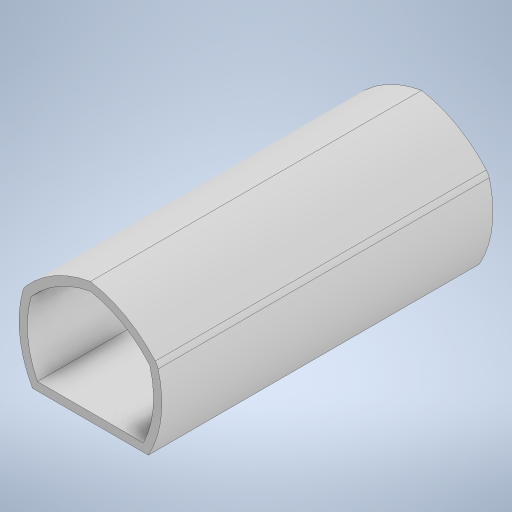
# Autodesk Inventor part: body
Saved by Autodesk Inventor 2024 (Build 280153000, 153)
## iProperties
Created: 2023-06-07
Part Number: body
Material: Generic
Document SubType Name: Modeling
Designer: tamiz
Density: 1 g/cm^3
Appearance: Default
Author: tamiz
Autodesk Inventor part; units mm, degrees
ref_plane "YZ Plane" through (0, 0, 0) normal (1, 0, 0) x (0, 1, 0)
ref_plane "XZ Plane" through (0, 0, 0) normal (0, 1, 0) x (-1, 0, 0)
ref_plane "XY Plane" through (0, 0, 0) normal (0, 0, 1) x (1, 0, 0)
sketch "Sketch3" plane through (0, 0, 0) normal (0, 0, 1) x (1, 0, 0)
  line L0 (3200.4, -3619.5) -> (-3200.4, -3619.5)
  line L1 (0, -3619.5) -> (0, 3086.1) construction
  arc A0 (-3738.1541, 769.8538) -> (-3200.4, -3619.5) centre (1884.0877, -768.9648) ccw
  arc A1 (0, 3086.1) -> (-3578.7308, 1068.0837) centre (1038.9488, -2938.6136) ccw
  arc A2 (-3578.7308, 1068.0837) -> (-3738.1541, 769.8538) centre (-3003.1863, 568.6916) ccw
  arc A3 (3200.4, -3619.5) -> (3738.1541, 769.8538) centre (-1884.0877, -768.9648) ccw
  arc A4 (3578.7308, 1068.0837) -> (0, 3086.1) centre (-1038.9488, -2938.6136) ccw
  arc A5 (3738.1541, 769.8538) -> (3578.7308, 1068.0837) centre (3003.1863, 568.6916) ccw
  arc A6 (-3278.4432, 715.8952) -> (-2925.1203, -3162.3) centre (1884.0877, -768.9648) ccw
  line L2 (-2925.1203, -3162.3) -> (2925.1203, -3162.3)
  arc A7 (2925.1203, -3162.3) -> (3278.4432, 715.8952) centre (-1884.0877, -768.9648) ccw
  arc A8 (3278.4432, 715.8952) -> (0, 2621.5927) centre (-1038.9488, -2938.6136) ccw
  arc A9 (0, 2621.5927) -> (-3278.4432, 715.8952) centre (1038.9488, -2938.6136) ccw
  dimension "d3" = 6400.8
  dimension "d4" = 6705.6
  dimension "d5" = 762
  dimension "d6" = 457.2
  constraints: 20 point on circle, 10 centre point, 6 end point, 5 symmetric about line, 2 tangent, 1 midpoint, 1 vertical, 7 other
  measures "d3" distance of L0.start L0.end
  measures "d4" distance of L1.start L1.end
  measures "d5" radius of A2
  measures "d6" radial gap between concentric circles of A1 A9
extrude "Extrusion1" add sketch "Sketch3" against normal blind 18288
body "Solid1"
